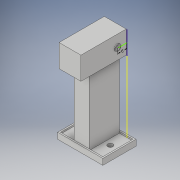
# Autodesk Inventor part: detector curvament fil
Saved by Autodesk Inventor 2019 (Build 230136000, 136)
## iProperties
Created: 2018-08-06
Part Number: detector curvament fil
Material: Genérico
Document SubType Name: Modeling
Designer: Albert Garangou Culebras
Density: 1 g/cm^3
Appearance: Valor por defecto
Mass: 54.1896 g
Surface Area: 120.446 cm^2
Volume: 54.1896 cm^3
Author: Albert Garangou Culebras
Title: suport detector curvament fil
Comments: Falta fer una possible guia per amagar el cable (dins la paret o a fora).
Autodesk Inventor part; units mm, degrees
ref_plane "YZ Plane" through (0, 0, 0) normal (1, 0, 0) x (0, 1, 0)
ref_plane "XZ Plane" through (0, 0, 0) normal (0, 1, 0) x (-1, 0, 0)
ref_plane "XY Plane" through (0, 0, 0) normal (0, 0, 1) x (1, 0, 0)
sketch "base" plane through (0, 0, 0) normal (0, 1, 0) x (-1, 0, 0)
  line L0 (0, 0) -> (0, -20)
  line L1 (0, -20) -> (10, -20)
  line L2 (10, -20) -> (10, 0)
  line L3 (10, 0) -> (0, 0)
  dimension "d186" = 20
  dimension "d187" = 10
  constraints: 8 end point, 3 perpendicular, 1 vertical
  measures "d186" distance of L0.start L0.end
  measures "d187" distance of L0.end L1.end
extrude "Extrusión29" add sketch "base" along normal blind 50
sketch "Boceto41" plane through (0, 50, 0) normal (0, 1, 0) x (1, 0, 0)
  line L0 (0, 20) -> (5, 20)
  line L1 (5, 20) -> (5, 0)
  line L2 (-10, 0) -> (0, 0) projected
  line L3 (5, 0) -> (-10, 0)
  line L4 (-10, 0) -> (-10, 20)
  line L5 (-10, 20) -> (5, 20)
  dimension "d190" = 5
  constraints: 10 end point, 2 collinear, 2 perpendicular, 1 horizontal, 1 point on line
  measures "d190" distance of L0.start L0.end
extrude "Extrusión30" add sketch "Boceto41" along normal blind 15
sketch "Boceto42" plane through (-10, 0, 0) normal (0, 0, 1) x (1, 0, 0)
  line L0 (15, 50) -> (10, 50) projected
  line L1 (15, 50) -> (0, 50)
  line L2 (0, 0) -> (0, 65) projected
  line L3 (0, 50) -> (0, 65)
  line L4 (0, 65) -> (15, 65) projected
  line L5 (0, 65) -> (15, 65)
  line L6 (15, 65) -> (15, 50)
  point P0 (10, 0)
  constraints: 8 end point, 2 perpendicular, 1 collinear, 1 horizontal
extrude "Extrusión31" add sketch "Boceto42" along normal blind 10
sketch "Boceto45" plane through (5, 50, -20) normal (1, 0, 0) x (0, 0, -1)
  line L0 (0, -50) -> (0, 15) projected
  line L1 (0, 0) -> (0, 15)
  line L2 (0, 7.5) -> (-6, 7.5)
  point P0 (-20, -50)
  dimension "d200" = 6
  constraints: 4 end point, 1 collinear, 1 horizontal, 1 midpoint
  measures "d200" distance of L2.start L2.end
hole "Agujero1" at (5, 57.5, -14) direction (-1, 0, 0) diameter 3.2 end through all
sketch "Boceto51" plane through (-10, 0, -20) normal (-1, 0, 0) x (0, 0, 1)
  circle A0 centre (6, 57.5) radius 1.6 projected
  circle A1 centre (6, 57.5) radius 1.6
  point P0 (20, 0)
  constraints: 1 centre point, 1 coincident
hole "Agujero2" at (-10, 57.5, -14) direction (1, 0, 0) diameter 3.2 depth 30 counterbore diameter 10 counterbore depth 5
sketch "Boceto52" plane through (0, 0, 0) normal (0, -1, 0) x (1, 0, 0)
  line L0 (0, 0) -> (0, -20) projected
  line L1 (10, 0) -> (10, -20)
  line L2 (-10, 0) -> (0, 0) projected
  line L3 (-20, 0) -> (-20, -20)
  line L4 (-20, -20) -> (-20, -21)
  line L5 (-20, 0) -> (-20, 1)
  line L6 (10, 0) -> (10, 1)
  line L7 (10, -20) -> (10, -21)
  line L8 (10, -21) -> (-20, -21)
  line L9 (10, 1) -> (-20, 1)
  dimension "d237" = 10
  dimension "d238" = 20
  dimension "d239" = 10
  dimension "d240" = 20
  dimension "d241" = 1
  dimension "d242" = 1
  dimension "d244" = 1
  constraints: 16 end point, 3 vertical, 1 point on line
  measures "d237" distance of L0.start L1.start
  measures "d238" distance of L1.start L1.end
  measures "d239" distance of L2.start L3.start
  measures "d240" distance of L3.start L3.end
  measures "d241" distance of L3.end L4.end
  measures "d242" distance of L3.start L5.end
  measures "d244" distance of L1.end L7.end
extrude "Extrusión36" add sketch "Boceto52" against normal blind 3
sketch "Boceto53" plane through (0, 3, 0) normal (0, 1, 0) x (1, 0, 0)
  line L0 (-20, 21) -> (-20, -1) projected
  line L1 (-19, 0) -> (-19, 20)
  line L2 (-19, 20) -> (9, 20)
  line L3 (9, 20) -> (9, 0)
  line L4 (9, 0) -> (-19, 0)
  line L5 (-20, 21) -> (-20, -1) projected
  line L6 (10, -1) -> (10, 21) projected
  line L7 (-20, -1) -> (10, -1)
  line L8 (10, -1) -> (10, 21)
  line L9 (10, 21) -> (-20, 21)
  line L10 (-20, 21) -> (-20, -1)
  point P0 (0, 0)
  dimension "d248" = 20
  dimension "d249" = 28
  dimension "d250" = 20
  constraints: 16 end point, 2 parallel, 2 perpendicular, 1 horizontal
  measures "d248" distance of L1.start L1.end
  measures "d249" distance of L1.end L2.end
  measures "d250" distance of L2.end L3.end
extrude "Extrusión37" add sketch "Boceto53" along normal blind 1
sketch "Boceto54" plane through (0, 3, 0) normal (0, 1, 0) x (1, 0, 0)
  circle A0 centre (-14, 10) radius 1.7
  circle A1 centre (4, 10) radius 1.7
  dimension "d259" = 3.4
  dimension "d261" = 3.4
  constraints: 2 centre point
  measures "d259" diameter of A0
  measures "d261" diameter of A1
extrude "Extrusión38" cut sketch "Boceto54" against normal blind 39
sketch "Boceto55" plane through (5, 50, -20) normal (1, 0, 0) x (0, 0, -1)
  line L0 (-30, 15) -> (-30, 0) projected
  line L1 (0, 15) -> (-30, 15)
  line L2 (-30, 15) -> (-30, 0)
  line L3 (-30, 0) -> (0, 0)
  line L4 (0, 0) -> (0, 15)
  circle A0 centre (-6, 7.5) radius 1.6
  circle A1 centre (-6, 7.5) radius 2.1
  point P0 (-20, -50)
  dimension "d264" = 4.2
  constraints: 8 end point, 2 centre point, 2 parallel, 1 coincident, 1 horizontal, 1 perpendicular
  measures "d264" diameter of A1
extrude "Extrusión39" cut sketch "Boceto55" against normal blind 0.5 contours L1 L4 L3 L0
